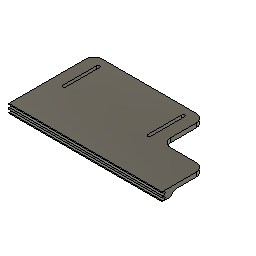
rakel v4 v1 (Autodesk Fusion 360 design; units mm, degrees)
Autodesk Fusion 360 part; units mm, degrees
note: some values were not read from the file. Set by a fixed rule: which sketch regions a step uses.
sketch "Skizze1" plane through (0, 0, 0) normal (0, 0, 1) x (1, 0, 0)
  line L0 (0, 0) -> (180, 0)
  line L1 (180, 0) -> (180, 40)
  line L2 (120, 100) -> (10, 100)
  line L3 (0, 90) -> (0, 0)
  line L4 (115, 100) -> (115, 50) construction
  line L5 (15, 100) -> (15, 50) construction
  circle A0 centre (15, 50) radius 1.75
  circle A1 centre (115, 50) radius 1.75
  circle A2 centre (15, 90) radius 1.75
  circle A3 centre (115, 90) radius 1.75
  line L6 (13.25, 50) -> (13.25, 90)
  line L7 (16.75, 90) -> (16.75, 50)
  line L8 (113.25, 90) -> (113.25, 50)
  line L9 (116.75, 50) -> (116.75, 90)
  line L10 (130, 90) -> (130, 60)
  line L11 (140, 50) -> (170, 50)
  line L12 (130, 50) -> (170, 50)
  arc A4 (130, 90) -> (120, 100) centre (120, 90) ccw
  arc A5 (10, 100) -> (0, 90) centre (10, 90) ccw
  arc A6 (130, 60) -> (140, 50) centre (140, 60) ccw
  arc A7 (180, 40) -> (170, 50) centre (170, 40) ccw
  point P0 (0, 100)
  dimension "d1" = 180
  dimension "d2" = 100
  dimension "d6" = 3.5
  dimension "d7" = 3.5
  dimension "d8" = 3.5
  dimension "d9" = 3.5
  dimension "d10" = 10
  dimension "d11" = 10
  dimension "d12" = 10
  constraint horizontal L0
  constraint vertical L1
  constraint horizontal L2
  constraint vertical L3
  constraint coincident L0.start L3.end
  constraint coincident L2 L4.start
  constraint coincident L2 L5.start
  constraint perpendicular L2 L5
  constraint coincident L5.end A0.centre
  constraint coincident L4.end A1.centre
  constraint coincident L5 A2.centre
  constraint coincident L4 A3.centre
  constraint coincident A0 L6.start
  constraint coincident A2 L6.end
  constraint tangent A2 L6
  constraint parallel L5 L6
  constraint coincident A2 L7.start
  constraint coincident A0 L7.end
  constraint tangent A0 L7
  constraint parallel L5 L7
  constraint coincident A3 L8.start
  constraint coincident A1 L8.end
  constraint tangent A1 L8
  constraint parallel L4 L8
  constraint coincident A1 L9.start
  constraint coincident A3 L9.end
  constraint tangent A3 L9
  constraint parallel L4 L9
  constraint perpendicular L2 L10
  constraint tangent L10 A4
  constraint tangent L2 A4
  constraint coincident P0 L2
  constraint coincident P0 L3
  constraint tangent L2 A5
  constraint tangent L3 A5
  constraint coincident L12.start L11
  constraint coincident L12.start L10
  constraint tangent L11 A6
  constraint tangent L10 A6
  constraint tangent L1 A7
  constraint tangent L12 A7
  constraint equal A6 A7
  measures "d1" distance of L0.start L0.end
  measures "d2" distance of L0.start P0
  measures "d6" diameter of A0
  measures "d7" diameter of A1
  measures "d8" diameter of A2
  measures "d9" diameter of A3
  measures "d10" radius of A4
  measures "d11" radius of A5
  measures "d12" radius of A6
extrude "Extrusion1" add sketch "Skizze1" along normal blind 5
sketch "Skizze2" plane through (0, 0, 5) normal (0, 0, 1) x (-1, 0, 0)
  arc A0 (-13.25, -50) -> (-16.75, -50) centre (-15, -50) ccw
  line L0 (-13.25, -50) -> (-13.25, -90)
  arc A1 (-16.75, -90) -> (-13.25, -90) centre (-15, -90) ccw
  line L1 (-16.75, -90) -> (-16.75, -50)
  line L2 (-116.75, -90) -> (-116.75, -50)
  arc A2 (-113.25, -50) -> (-116.75, -50) centre (-115, -50) ccw
  line L3 (-113.25, -50) -> (-113.25, -90)
  arc A3 (-116.75, -90) -> (-113.25, -90) centre (-115, -90) ccw
  arc A4 (-130, -90) -> (-120, -100) centre (-120, -90) ccw
  line L4 (-120, -100) -> (-10, -100)
  arc A5 (-10, -100) -> (0, -90) centre (-10, -90) ccw
  line L5 (0, -90) -> (0, 0)
  line L6 (0, 0) -> (-180, 0)
  line L7 (-180, 0) -> (-180, -40)
  arc A6 (-180, -40) -> (-170, -50) centre (-170, -40) ccw
  line L8 (-170, -50) -> (-140, -50)
  arc A7 (-130, -60) -> (-140, -50) centre (-140, -60) ccw
  line L9 (-130, -60) -> (-130, -90)
  line L10 (0, 0) -> (0, -10)
  line L11 (0, -10) -> (-180, -10)
  line L12 (-180, -10) -> (-180, 0)
  line L13 (-180, 0) -> (0, 0)
  constraint coincident L5.end L6.start
  constraint coincident L5 L10.end
  constraint perpendicular L6 L10
  constraint coincident L7 L11.end
  constraint perpendicular L7 L11
  constraint coincident L6.end L7.start
extrude "Extrusion2" add sketch "Skizze2" against normal blind 10 contours L5 L6 L7 L10 L11 L12 L13
sketch "Skizze3" plane through (180, 0, 0) normal (1, 0, 0) x (0, 1, 0)
  line L0 (10, 0) -> (40, 0)
  line L1 (40, 0) -> (40, 5)
  line L2 (40, 5) -> (0, 5)
  line L3 (0, 5) -> (0, -5)
  line L4 (0, -5) -> (10, -5)
  line L5 (10, -5) -> (10, 0)
  circle A0 centre (1.5, 2.5) radius 2
  circle A1 centre (1.5, -2.5) radius 2
  dimension "d17" = 4
  dimension "d18" = 4
  measures "d17" diameter of A0
  measures "d18" diameter of A1
extrude "Extrusion3" cut sketch "Skizze3" against normal blind 197 contours L3 A1 | L3 A0 picked at (1.2641, -3.0074) picked at (0.6207, 3.1043)
fillet "Abrundung1" radius 10 1 edges at (90, 10, 0)
